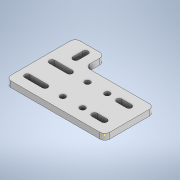
# Autodesk Inventor part: X_Carriage_Plate
Saved by Autodesk Inventor 2021 (Build 250183000, 183)
## iProperties
Created: 2021-06-13
Part Number: X_Carriage_Plate
Material: Generic
Document SubType Name: Modeling
Designer: Jorian Brusind
Density: 1 g/cm^3
Appearance: Default
Author: Jorian Brusind
Autodesk Inventor part; units mm, degrees
ref_plane "YZ Plane" through (0, 0, 0) normal (1, 0, 0) x (0, 1, 0)
ref_plane "XZ Plane" through (0, 0, 0) normal (0, 1, 0) x (-1, 0, 0)
ref_plane "XY Plane" through (0, 0, 0) normal (0, 0, 1) x (1, 0, 0)
sketch "Sketch1" plane through (0, 0, 0) normal (0, 1, 0) x (-1, 0, 0)
  line L0 (0, 0) -> (100, 0)
  line L1 (100, 0) -> (100, -50)
  line L2 (100, -50) -> (0, -50)
  line L3 (0, -50) -> (0, 0)
  line L4 (0, 0) -> (0, -16.6667)
  line L5 (0, -16.6667) -> (6, -16.6667)
  dimension "d0" = 100
  dimension "d1" = 50
  dimension "d2" = 16.6667
  dimension "d3" = 6
  constraints: 12 end point, 2 parallel, 2 perpendicular, 1 horizontal, 1 point on line
  measures "d0" distance of L1.end L2.end
  measures "d1" distance of L0.end L1.end
  measures "d2" distance of L0.start L4.end
  measures "d3" distance of L4.end L5.end
extrude "Extrusion1" add sketch "Sketch1" along normal blind 6
sketch "Sketch3" plane through (0, 6, 0) normal (0, 1, 0) x (1, 0, 0)
  circle A0 centre (-13, 12.5) radius 2.75
  line L0 (0, 0) -> (0, 50) projected
  line L1 (-100, 0) -> (0, 0) projected
  circle A1 centre (-13, 37.5) radius 2.75
  line L2 (-13, 12.5) -> (-18, 12.5)
  line L3 (-23, 12.5) -> (-13, 12.5) construction
  line L4 (-23, 9.75) -> (-13, 9.75)
  line L5 (-13, 15.25) -> (-23, 15.25)
  arc A2 (-23, 15.25) -> (-23, 9.75) centre (-23, 12.5) ccw
  arc A3 (-13, 9.75) -> (-13, 15.25) centre (-13, 12.5) ccw
  line L6 (-13, 37.5) -> (-18, 37.5)
  line L7 (-13, 37.5) -> (-8, 37.5) construction
  line L8 (-23, 37.5) -> (-13, 37.5) construction
  line L9 (-23, 34.75) -> (-13, 34.75)
  line L10 (-13, 40.25) -> (-23, 40.25)
  arc A4 (-23, 40.25) -> (-23, 34.75) centre (-23, 37.5) ccw
  arc A5 (-13, 34.75) -> (-13, 40.25) centre (-13, 37.5) ccw
  dimension "d21" = 5.5
  dimension "d22" = 13
  dimension "d23" = 12.5
  dimension "d26" = 25
  dimension "d87" = 5
  dimension "d88" = 5
  dimension "d89" = 180
  constraints: 22 end point, 8 point on circle, 8 tangent, 6 centre point, 4 horizontal, 2 collinear, 2 concentric, 2 midpoint, 2 parallel, 1 vertical, 2 other
  measures "d21" diameter of A0
  measures "d22" distance from line of L0 L2.start
  measures "d23" distance from line of L1 L2.start
  measures "d26" distance of L2.start L6.start
  measures "d87" distance of L2.start L2.end
  measures "d88" distance of L6.start L6.end
  measures "d89" angle of L6 L7
extrude "Extrusion3" cut sketch "Sketch3" against normal through all
sketch "Sketch4" plane through (0, 6, 0) normal (0, 1, 0) x (1, 0, 0)
  arc A0 (-13, 9.75) -> (-13, 15.25) centre (-13, 12.5) ccw projected
  line L0 (-13, 12.5) -> (-73, 12.5)
  line L1 (-73, 12.5) -> (-91, 12.5) construction
  line L2 (-73, 15.25) -> (-91, 15.25)
  line L3 (-91, 9.75) -> (-73, 9.75)
  arc A1 (-73, 9.75) -> (-73, 15.25) centre (-73, 12.5) ccw
  arc A2 (-91, 15.25) -> (-91, 9.75) centre (-91, 12.5) ccw
  point P0 (0, 0)
  point P1 (-82, 12.5)
  dimension "d33" = 60
  dimension "d34" = 18
  dimension "d35" = 5.5
  constraints: 10 end point, 4 point on circle, 4 tangent, 2 centre point, 2 horizontal, 1 midpoint, 1 parallel
  measures "d33" distance of L0.start L0.end
  measures "d34" distance of L0.end L1.end
  measures "d35" diameter of A2
extrude "Extrusion4" cut sketch "Sketch4" against normal through all
pattern_linear "Rectangular Pattern2" count 2 spacing 25 along (0, 0, -1) of "Extrusion4"
sketch "Sketch5" plane through (0, 0, -50) normal (0, 0, -1) x (-1, 0, 0)
  line L0 (100, 0) -> (100, 6) projected
  line L1 (100, 0) -> (0, 0) projected
  line L2 (100, 6) -> (70, 6)
  line L3 (70, 6) -> (70, 0)
  line L4 (70, 0) -> (100, 0)
  line L5 (100, 0) -> (100, 6)
  dimension "d45" = 30
  constraints: 8 end point, 2 parallel, 1 horizontal, 1 perpendicular, 1 point on line
  measures "d45" distance of L4.end L3.end
extrude "Extrusion5" add sketch "Sketch5" along normal blind 20
sketch "Sketch6" plane through (0, 6, 0) normal (0, 1, 0) x (1, 0, 0)
  line L0 (-82, 52.5) -> (-82, 62.5) construction
  line L1 (-79.25, 52.5) -> (-79.25, 62.5)
  line L2 (-84.75, 62.5) -> (-84.75, 52.5)
  arc A0 (-84.75, 52.5) -> (-79.25, 52.5) centre (-82, 52.5) ccw
  arc A1 (-79.25, 62.5) -> (-84.75, 62.5) centre (-82, 62.5) ccw
  line L3 (-70, 50) -> (-70, 70) projected
  arc A2 (-91, 40.25) -> (-91, 34.75) centre (-91, 37.5) ccw projected
  point P0 (0, 0)
  point P1 (-82, 57.5)
  dimension "d48" = 10
  dimension "d49" = 5.5
  dimension "d50" = 12
  dimension "d51" = 20
  constraints: 8 end point, 4 point on circle, 4 tangent, 2 centre point, 1 midpoint, 1 parallel, 1 vertical
  measures "d48" distance of L0.start L0.end
  measures "d49" diameter of A1
  measures "d50" distance from line of L3 point (-82, 57.5)
  measures "d51" vertical distance of A2.centre point (-82, 57.5)
extrude "Extrusion6" cut sketch "Sketch6" against normal through all
fillet "Fillet2" radius 5 6 edges at (-100, 3, 0) (0, 3, 0) (-70, 3, -70) (-100, 3, -70) (0, 3, -50) (-70, 3, -50)
sketch "Sketch7" plane through (0, 6, 0) normal (0, 1, 0) x (1, 0, 0)
  arc A0 (-13, 9.75) -> (-13, 15.25) centre (-13, 12.5) ccw projected
  line L0 (-13, 12.5) -> (-35, 12.5)
  line L1 (-35, 12.5) -> (-55, 12.5)
  circle A1 centre (-55, 12.5) radius 2.75
  circle A2 centre (-35, 12.5) radius 2.75
  line L2 (0, 5) -> (0, 45) projected
  line L3 (0, 0) -> (0, 45)
  circle A3 centre (-35, 37.5) radius 2.75
  circle A4 centre (-55, 37.5) radius 2.75
  dimension "d55" = 22
  dimension "d56" = 20
  dimension "d57" = 5.5
  dimension "d58" = 5.5
  dimension "d61" = 25
  constraints: 6 end point, 4 centre point, 2 coincident, 2 horizontal, 1 collinear, 1 vertical, 4 other
  measures "d55" distance of L0.start L0.end
  measures "d56" distance of L0.end L1.end
  measures "d57" diameter of A1
  measures "d58" diameter of A2
  measures "d61" distance of A2.centre A3.centre
extrude "Extrusion7" cut sketch "Sketch7" against normal through all
sketch "Sketch9" plane through (0, 6, 0) normal (0, 1, 0) x (1, 0, 0)
  point P0 (0, 0)
body "Solid1"
